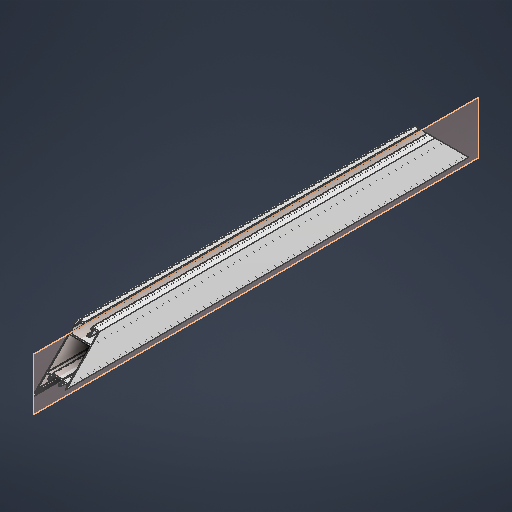
# Autodesk Inventor part: SP40-02 HOJA PUERTA BATIENTE INT - EXT
Saved by Autodesk Inventor 2025 (Build 290162000, 162)
## iProperties
Created: 2026-01-18
Part Number: SP40-02 HOJA PUERTA BATIENTE INT - EXT
Material: Aluminio
Document SubType Name: Modeling
Designer: ROLANDO
Density: 2.7 g/cm^3
Appearance: Satinado
Author: ROLANDO
Autodesk Inventor part; units mm, degrees
ref_plane "YZ Plane" through (0, 0, 0) normal (1, 0, 0) x (0, 1, 0)
ref_plane "XZ Plane" through (0, 0, 0) normal (0, 1, 0) x (-1, 0, 0)
sketch "Boceto1" plane through (0, 0, 0) normal (0, 0, 1) x (1, 0, 0)
  line L0 (37.5, 0.5) -> (37.5, 38.8)
  line L1 (37, 39.3) -> (0.5, 39.3)
  line L2 (0, 38.8) -> (0, 0.5)
  line L3 (0.5, 40.7) -> (37, 40.7)
  line L4 (38.9, 55.1) -> (38.9, -5.3)
  line L5 (-1.4, -22.9) -> (-1.4, 50.96)
  line L6 (37.5, 41.2) -> (37.5, 53.7)
  line L7 (38.9, 55.1) -> (24.7, 55.1)
  line L8 (24.7, 55.1) -> (24.7, 53.46)
  line L9 (28.5, 53.7) -> (28.5, 47.2)
  line L10 (29.9, 45.8) -> (29.9, 53.7)
  line L11 (29.9, 45.8) -> (24.7, 45.8)
  line L12 (24.7, 45.8) -> (24.7, 47.44)
  line L13 (26.1, 47.2) -> (28.5, 47.2)
  line L14 (26.1, 48.45) -> (25.3942, 48.45)
  line L15 (25.3942, 48.45) -> (24.7, 47.44)
  line L16 (26.1, 52.45) -> (25.3942, 52.45)
  line L17 (0, 41.2) -> (0, 48.2)
  line L18 (0, 48.2) -> (1.5, 48.2)
  line L19 (1.5, 48.2) -> (1.5, 50.96)
  line L20 (2.74, 55.1) -> (10.9, 55.1)
  line L21 (9.4619, 53.7) -> (4.24, 53.7)
  line L22 (10.9, 55.1) -> (10.9, 52.6)
  line L23 (10.9, 52.6) -> (10.19, 52.6)
  line L24 (10.19, 52.6) -> (9.4619, 53.7)
  line L25 (0, -24.4) -> (0.1, -24.4)
  line L26 (37.5, -1.9) -> (37.5, -5.3)
  line L27 (38, -5.8) -> (38.4, -5.8)
  line L28 (26.9, -1.4) -> (26.9, -4.4)
  line L29 (28.3, -5.8) -> (28.3, -1.9)
  line L30 (5.5, -1.9) -> (5.5, -5.8)
  line L31 (6.9, -4.4) -> (6.9, -1.4)
  line L32 (6.9, -4.4) -> (9.4, -4.4)
  line L33 (9.4, -4.4) -> (9.4, -5.8)
  line L34 (9.4, -5.8) -> (5.5, -5.8)
  line L35 (26.9, -4.4) -> (24.4, -4.4)
  line L36 (24.4, -4.4) -> (24.4, -5.8)
  line L37 (24.4, -5.8) -> (28.3, -5.8)
  line L38 (25.8, 0.5) -> (25.8, 1.4)
  line L39 (25.8, 1.4) -> (8, 1.4)
  line L40 (0.5, 0) -> (7.5, 0)
  line L41 (26.3, 0) -> (37, 0)
  line L42 (24.4, -1.4) -> (24.4, 0)
  line L43 (9.4, 0) -> (9.4, -1.4)
  line L44 (26.1, 53.7) -> (28.5, 53.7)
  line L45 (29.9, 53.7) -> (37.5, 53.7)
  line L46 (37, -1.4) -> (28.8, -1.4)
  line L47 (9.4, -1.4) -> (6.9, -1.4)
  line L48 (5, -1.4) -> (0, -1.4)
  arc A0 (4.24, 53.7) -> (1.5, 50.96) centre (4.24, 50.96) ccw
  arc A1 (2.74, 55.1) -> (-1.4, 50.96) centre (2.74, 50.96) ccw
  line L49 (26.9, -1.4) -> (24.4, -1.4)
  line L50 (26.9, -1.4) -> (24.4, -1.4)
  line L51 (8, 1.4) -> (8, 0.5)
  line L52 (9.4, 0) -> (24.4, 0)
  line L53 (24.7, 53.46) -> (25.3942, 52.45)
  line L54 (26.1, 53.7) -> (26.1, 52.45)
  line L55 (26.1, 47.2) -> (26.1, 48.45)
  line L56 (0, -24.4) -> (1, -24.4)
  line L57 (0.6, -23) -> (0.5, -23)
  line L58 (0.5, -17.8) -> (0.6, -17.8)
  line L59 (1, -16.4) -> (0, -16.4)
  line L60 (1.1, -18.3) -> (1.1, -18.4)
  line L61 (1.6, -18.9) -> (2, -18.9)
  line L62 (2.5, -18.4) -> (2.5, -17.9)
  line L63 (1.1, -22.5) -> (1.1, -22.4)
  line L64 (1.6, -21.9) -> (2, -21.9)
  line L65 (2.5, -22.4) -> (2.5, -22.9)
  line L66 (0, -1.4) -> (0, -16.4)
  line L67 (0, -18.3) -> (0, -22.5)
  arc A2 (2.5, -17.9) -> (1, -16.4) centre (1, -17.9) ccw
  arc A3 (1, -24.4) -> (2.5, -22.9) centre (1, -22.9) ccw
  arc A4 (-1.4, -22.9) -> (0.1, -24.4) centre (0.1, -22.9) ccw
  arc A5 (1.1, -18.4) -> (1.6, -18.9) centre (1.6, -18.4) ccw
  arc A6 (1.1, -18.3) -> (0.6, -17.8) centre (0.6, -18.3) ccw
  arc A7 (2, -18.9) -> (2.5, -18.4) centre (2, -18.4) ccw
  arc A8 (2.5, -22.4) -> (2, -21.9) centre (2, -22.4) ccw
  arc A9 (1.6, -21.9) -> (1.1, -22.4) centre (1.6, -22.4) ccw
  arc A10 (0.6, -23) -> (1.1, -22.5) centre (0.6, -22.5) ccw
  arc A11 (5.5, -1.9) -> (5, -1.4) centre (5, -1.9) ccw
  arc A12 (7.5, 0) -> (8, 0.5) centre (7.5, 0.5) ccw
  arc A13 (0, 0.5) -> (0.5, 0) centre (0.5, 0.5) ccw
  arc A14 (28.8, -1.4) -> (28.3, -1.9) centre (28.8, -1.9) ccw
  arc A15 (25.8, 0.5) -> (26.3, 0) centre (26.3, 0.5) ccw
  arc A16 (37, 0) -> (37.5, 0.5) centre (37, 0.5) ccw
  arc A17 (37.5, -1.9) -> (37, -1.4) centre (37, -1.9) ccw
  arc A18 (37.5, -5.3) -> (38, -5.8) centre (38, -5.3) ccw
  arc A19 (38.4, -5.8) -> (38.9, -5.3) centre (38.4, -5.3) ccw
  arc A20 (0.5, 39.3) -> (0, 38.8) centre (0.5, 38.8) ccw
  arc A21 (37.5, 38.8) -> (37, 39.3) centre (37, 38.8) ccw
  arc A22 (37, 40.7) -> (37.5, 41.2) centre (37, 41.2) ccw
  arc A23 (0, 41.2) -> (0.5, 40.7) centre (0.5, 41.2) ccw
  arc A24 (0, -22.5) -> (0.5, -23) centre (0.5, -22.5) ccw
  arc A25 (0.5, -17.8) -> (0, -18.3) centre (0.5, -18.3) ccw
  point P0 (0, 0)
  point P1 (9.4, -5.1)
  point P2 (27.3, 45.8)
  point P3 (28.5, 50.45)
  point P4 (0, -23)
  point P5 (0, -17.8)
  point P6 (1.1, -21.9)
  point P7 (0, -20.4)
  dimension "d10" = 60.9
  dimension "d11" = 23
  dimension "d13" = 39.3
  dimension "d14" = 1.4
  dimension "d15" = 1.4
  dimension "d17" = 1.4
  dimension "d18" = 1.4
  dimension "d20" = 1.4
  dimension "d22" = 1.4
  dimension "d23" = 1.4
  dimension "d26" = 1.4
  dimension "d27" = 1.4
  dimension "d28" = 1.4
  dimension "d31" = 1.4
  dimension "d34" = 40.3
  dimension "d35" = 37.9
  dimension "d36" = 39.3
  dimension "d37" = 37.5
  dimension "d38" = 37.5
  dimension "d40" = 14.2
  dimension "d41" = 13.8
  dimension "d42" = 2.5
  dimension "d43" = 0.71
  dimension "d45" = 2.9
  dimension "d46" = 14.4
  dimension "d47" = 33.5
  dimension "d48" = 7.5
  dimension "d51" = 2.74
  dimension "d58" = 4.14
  dimension "d59" = 6.9
  dimension "d60" = 1.4
  dimension "d61" = 20
  dimension "d62" = 6.9
  dimension "d64" = 1.4
  dimension "d65" = 3
  dimension "d66" = 3
  dimension "d68" = 2.5
  dimension "d69" = 2.5
  dimension "d70" = 15
  dimension "d71" = 2.5
  dimension "d73" = 1.4
  dimension "d74" = 1.4
  dimension "d75" = 1.4
  dimension "d76" = 1.4
  dimension "d77" = 9.3
  dimension "d82" = 1.4
  dimension "d83" = 1.4
  dimension "d84" = 1.4
  dimension "d85" = 1.4
  dimension "d86" = 1.4
  dimension "d88" = 2.4
  dimension "d95" = 6.02
  dimension "d99" = 111
  dimension "d100" = 2.4
  dimension "d109" = 0.7058
  dimension "d110" = 0.7058
  dimension "d112" = 5.2
  dimension "d115" = 2.6
  dimension "d116" = 2.6
  dimension "d117" = 1.5
  dimension "d118" = 1.5
  dimension "d119" = 3
  dimension "d120" = 1.4
  dimension "d121" = 1.4
  constraints: 136 end point, 52 point on circle, 52 tangent, 26 centre point, 22 parallel, 20 equal radius, 15 horizontal, 14 perpendicular, 12 point on line, 5 vertical, 4 midpoint, 3 collinear, 2 equal length
  measures "d10" distance between parallel lines of L27 L7
  measures "d11" distance between parallel lines of L25 L48
  measures "d13" distance between parallel lines of L41 L1
  measures "d14" distance between parallel lines of L40 L48
  measures "d15" distance between parallel lines of L41 L46
  measures "d17" distance between parallel lines of L28 L29
  measures "d18" distance between parallel lines of L35 L37
  measures "d20" distance between parallel lines of L40 L47
  measures "d22" distance between parallel lines of L32 L34
  measures "d23" distance between parallel lines of L31 L30
  measures "d26" distance between parallel lines of L5 L2
  measures "d27" distance between parallel lines of L3 L1
  measures "d28" distance between parallel lines of L4 L6
  measures "d31" distance between parallel lines of L21 L20
  measures "d34" distance between parallel lines of L5 L4
  measures "d35" distance between parallel lines of L1 L39
  measures "d36" distance between parallel lines of L1 L40
  measures "d37" distance between parallel lines of L6 L17
  measures "d38" distance between parallel lines of L2 L0
  measures "d40" distance between parallel lines of L4 L8
  measures "d41" distance between parallel lines of L22 L8
  measures "d42" distance of L20.end L22.end
  measures "d43" distance of L22.end L23.end
  measures "d45" distance between parallel lines of L19 L5
  measures "d46" distance between parallel lines of L3 L7
  measures "d47" angle of L22 L24
  measures "d48" distance between parallel lines of L3 L18
  measures "d51" radius of A0
  measures "d58" radius of A1
  measures "d59" distance between parallel lines of L18 L20
  measures "d60" distance between parallel lines of L5 L17
  measures "d61" distance between parallel lines of L28 L31
  measures "d62" distance between parallel lines of L2 L31
  measures "d64" distance between parallel lines of L49 L41
  measures "d65" distance between parallel lines of L49 L35
  measures "d66" distance between parallel lines of L47 L32
  measures "d68" distance between parallel lines of L31 L43
  measures "d69" distance between parallel lines of L28 L42
  measures "d70" distance between parallel lines of L33 L36
  measures "d71" distance from line of L31 point (9.4, -5.1)
  measures "d73" distance between parallel lines of L51 L43
  measures "d74" distance between parallel lines of L38 L42
  measures "d75" distance between parallel lines of L4 L26
  measures "d76" distance between parallel lines of L4 L0
  measures "d77" distance between parallel lines of L11 L7
  measures "d82" distance between parallel lines of L10 L9
  measures "d83" distance from line of point (27.3, 45.8) L13
  measures "d84" distance between parallel lines of L12 L55
  measures "d85" distance between parallel lines of L8 L54
  measures "d86" distance between parallel lines of L7 L44
  measures "d88" distance between parallel lines of L9 L54
  measures "d95" distance of L12.end L8.end
  measures "d99" angle of L15 L53
  measures "d100" distance between parallel lines of L9 L55
  measures "d109" distance of L16.start L16.end
  measures "d110" distance of L14.start L14.end
  measures "d112" distance between parallel lines of L57 L58
  measures "d115" distance from line of point (0, -20.4) L58
  measures "d116" distance from line of point (0, -20.4) L57
  measures "d117" distance from line of point (0, -20.4) L61
  measures "d118" distance from line of point (0, -20.4) L64
  measures "d119" distance between parallel lines of L64 L61
  measures "d120" distance between parallel lines of L63 L65
  measures "d121" distance between parallel lines of L56 L57
extrude "Extrusión1" add sketch "Boceto1" against normal blind 761
ref_plane "Plano de trabajo1" through (0, 0, -380.5) normal (0, 0, 1) x (1, 0, 0)
sketch "Boceto2" plane through (38.9, -22.9, 0) normal (-1, 0, 0) x (0, 0, 1)
  line L0 (-761, -1.5) -> (-761, 78)
  line L1 (0, 1) -> (-761, 1) projected
  line L2 (0, -1.5) -> (-761, -1.5) projected
  line L3 (0, 78) -> (-761, 78) projected
  line L4 (-761, 78) -> (-681.5, 78)
  line L5 (-761, -1.5) -> (-681.5, 78)
  point P0 (-300.5, -1.5)
  dimension "d146" = 45
  constraints: 6 end point, 3 point on line, 1 vertical
  measures "d146" angle of L3 L5
extrude "Extrusión2" cut sketch "Boceto2" along normal up to surface (40.3 mm away)
mirror "Simetría2" about plane through (0, 0, -380.5) normal (0, 0, 1) of "Extrusión2"
ref_plane "Plano de trabajo2" through (18.75, -5.3, 0) normal (1, 0, 0) x (0, 0, -1)
